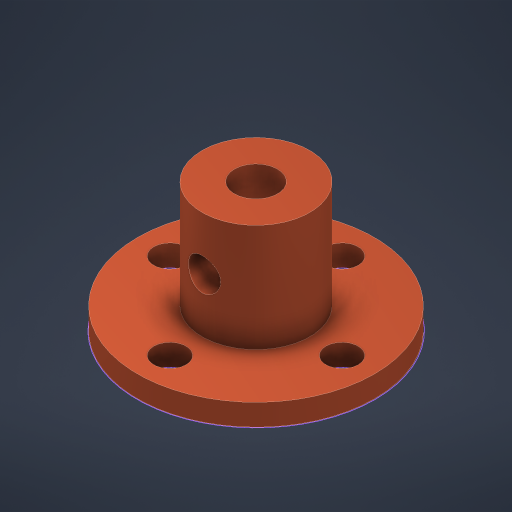
# Autodesk Inventor part: hub 4mm
Saved by Autodesk Inventor 2024.3 (Build 283343000, 343)
## iProperties
Created: 2025-06-12
Part Number: hub 4mm
Material: Copper
Document SubType Name: Modeling
Designer: Akbar Syihabuddin
Density: 8.94 g/cm^3
Appearance: Copper - Satin
Author: Akbar Syihabuddin
Autodesk Inventor part; units mm, degrees
ref_plane "YZ Plane" through (0, 0, 0) normal (1, 0, 0) x (0, 1, 0)
ref_plane "XZ Plane" through (0, 0, 0) normal (0, 1, 0) x (-1, 0, 0)
ref_plane "XY Plane" through (0, 0, 0) normal (0, 0, 1) x (1, 0, 0)
sketch "Sketch1" plane through (0, 0, 0) normal (0, 1, 0) x (-1, 0, 0)
  circle A0 centre (0, 0) radius 11
  circle A1 centre (0, 0) radius 5
  circle A2 centre (0, 0) radius 2
  line L0 (0, 0) -> (0, -8)
  line L1 (0, 0) -> (0, 8)
  circle A3 centre (0, 8) radius 1.5
  circle A4 centre (0, -8) radius 1.5
  circle A5 centre (-8, 0) radius 1.5
  circle A6 centre (0, -8) radius 1.5
  circle A7 centre (8, 0) radius 1.5
  dimension "d0" = 22
  dimension "d1" = 10
  dimension "d2" = 4
  dimension "d3" = 8
  dimension "d4" = 8
  dimension "d5" = 3
  dimension "d6" = 3
  dimension "d9" = 360
  constraints: 8 centre point, 5 coincident, 4 end point, 2 vertical, 9 other
  measures "d0" diameter of A0
  measures "d1" diameter of A1
  measures "d2" diameter of A2
  measures "d3" distance of L0.start L0.end
  measures "d4" distance of L0.start L1.end
  measures "d5" diameter of A3
  measures "d6" diameter of A4
extrude "Extrusion1" add sketch "Sketch1" along normal blind 2
extrude "Extrusion2" add sketch "Sketch1" along normal blind 12 contours A1 L0 A2 L1 | L1 A2 L0 A1
sketch "Sketch2" plane through (0, 0, 0) normal (0, 0, 1) x (1, 0, 0)
  circle A0 centre (0, 7.0307) radius 1.5
  point P0 (0, 0)
  dimension "d15" = 3
  constraints: 1 centre point
  measures "d15" diameter of A0
extrude "Extrusion3" cut sketch "Sketch2" along normal mid plane 12
sketch "Sketch3" plane through (0, 0, 0) normal (0, -1, 0) x (1, 0, 0)
  circle A0 centre (0, 0) radius 2
  circle A1 centre (-8, 0) radius 1.5 projected
  circle A2 centre (-8, 0) radius 1.5
  circle A3 centre (0, -8) radius 1.5 projected
  circle A4 centre (0, -8) radius 1.5
  circle A5 centre (8, 0) radius 1.5 projected
  circle A6 centre (8, 0) radius 1.5
  circle A7 centre (0, 8) radius 1.5 projected
  circle A8 centre (0, 8) radius 1.5
  circle A9 centre (0, 0) radius 11.0573
  constraints: 6 centre point, 6 coincident
body "Solid1"
